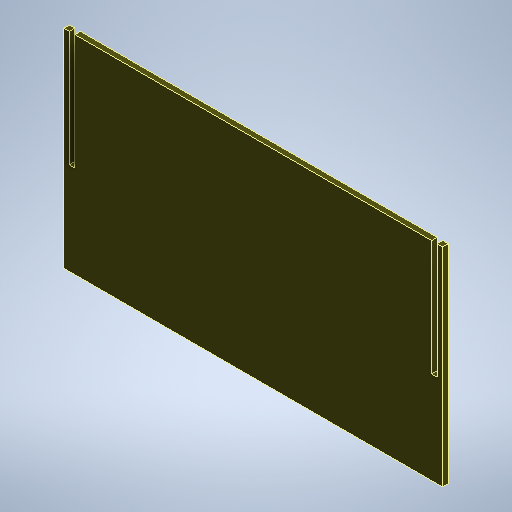
# Autodesk Inventor part: Finishing Sheets .2  ( Upper )
Saved by Autodesk Inventor 2025.4 (Build 294407000, 407)
## iProperties
Created: 2026-04-04
Part Number: Finishing Sheets .2  ( Upper )
Material: Generic
Document SubType Name: Sheet Metal
Designer: lenovo
Density: 1 g/cm^3
Sheet Metal Rule: Default_mm
Appearance: Default(2)
Author: lenovo
Autodesk Inventor part; units mm, degrees
ref_plane "YZ Plane" through (0, 0, 0) normal (1, 0, 0) x (0, 1, 0)
ref_plane "XZ Plane" through (0, 0, 0) normal (0, 1, 0) x (-1, 0, 0)
ref_plane "XY Plane" through (0, 0, 0) normal (0, 0, 1) x (1, 0, 0)
sketch "Sketch1" plane through (0, 0, 0) normal (0, 0, 1) x (1, 0, 0)
  line L0 (-102.5, -56.25) -> (102.5, -56.25)
  line L1 (102.5, -56.25) -> (102.5, 56.25)
  line L2 (102.5, 56.25) -> (-102.5, 56.25)
  line L3 (-102.5, 56.25) -> (-102.5, -56.25)
  line L4 (-102.5, -56.25) -> (102.5, 56.25) construction
  line L5 (102.5, -56.25) -> (-102.5, 56.25) construction
  line L6 (-20.5, 56.25) -> (20.5, 56.25)
  line L7 (20.5, 56.25) -> (20.5, 50.25)
  line L8 (20.5, 50.25) -> (-20.5, 50.25)
  line L9 (-20.5, 50.25) -> (-20.5, 56.25)
  point P0 (0, 0)
  point P1 (0, 56.25)
  point P2 (0, 56.25)
  point P3 (20.5, 56.25)
  dimension "d0" = 41
  dimension "d1" = 6
  dimension "d2" = 205
  dimension "d3" = 112.5
  measures "d0" distance of L7.end L8.end
  measures "d1" distance of L6.end L7.end
  measures "d2" distance of L1.end L2.end
  measures "d3" distance of L2.end L0.start
extrude "Plate1" add sketch "Sketch1" along normal blind 3
sketch "Sketch2" plane through (0, 0, 3) normal (0, 0, 1) x (1, 0, 0)
  line L0 (-102.5, 56.25) -> (102.5, 56.25) projected
  line L1 (-99.5, 56.25) -> (-96.5, 56.25)
  line L2 (-96.5, 56.25) -> (-96.5, -6.25)
  line L3 (-96.5, -6.25) -> (-99.5, -6.25)
  line L4 (-99.5, -6.25) -> (-99.5, 56.25)
  line L5 (-102.5, -56.25) -> (-102.5, 56.25) projected
  line L6 (102.5, -56.25) -> (-102.5, -56.25) projected
  point P0 (0, 0)
  point P1 (-20.5, 56.25)
  dimension "d5" = 3
  dimension "d6" = 3
  dimension "d8" = 50
  constraints: 8 end point, 2 parallel, 1 horizontal, 1 perpendicular, 1 point on line
  measures "d5" distance between parallel lines of L4 L2
  measures "d6" distance between parallel lines of L5 L4
  measures "d8" distance between parallel lines of L3 L6
extrude "Cut1" cut sketch "Sketch2" against normal blind 3
mirror "Mirror1" about plane through (0, 0, 0) normal (1, 0, 0) of "Cut1"
equation "\"d9\" = Thickness"
equation "\"d4\" = Thickness"
equation "\"BendRadius\" = Thickness"
equation "\"BendReliefWidth\" = Thickness"
equation "\"BendReliefDepth\" = 0.5 * Thickness"
equation "\"CornerReliefSize\" = 4 * Thickness"
equation "\"MinimumRemnant\" = 2 * Thickness"
equation "\"TransitionRadius\" = BendRadius"
equation "\"JacobiRadiusSize\" = BendRadius"
equation "\"GapSize\" = Thickness"
equation "\"Thickness\" = 3"
body "Solid1"
